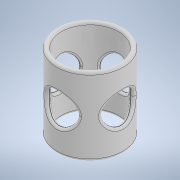
# Autodesk Inventor part: BlueYetiHolderSupport
Saved by Autodesk Inventor 2020 (Build 240168000, 168)
## iProperties
Created: 2020-08-02
Part Number: BlueYetiHolderSupport
Material: Generic
Document SubType Name: Sheet Metal
Designer: maple
Density: 1 g/cm^3
Sheet Metal Rule: Default
Appearance: Default
Author: maple
Autodesk Inventor part; units mm, degrees
ref_plane "YZ Plane" through (0, 0, 0) normal (1, 0, 0) x (0, 1, 0)
ref_plane "XZ Plane" through (0, 0, 0) normal (0, 1, 0) x (-1, 0, 0)
ref_plane "XY Plane" through (0, 0, 0) normal (0, 0, 1) x (1, 0, 0)
sketch "Sketch1" plane through (0, 0, 0) normal (0, 1, 0) x (-1, 0, 0)
  circle A0 centre (0, 0) radius 18.5
  line L0 (0, -18.5) -> (0, -21.5)
  circle A1 centre (0, 0) radius 21.5
  dimension "d0" = 37
  dimension "d1" = 3
  constraints: 2 coincident, 2 end point, 2 vertical alignment, 1 vertical, 4 other
  measures "d1" distance of L0.start L0.end
extrude "Extrusion1" add sketch "Sketch1" along normal blind 50
fillet "Fillet1" radius 1.5 4 edges at (18.5, 50, 0) (21.5, 50, 0) (18.5, 0, 0) (21.5, 0, 0)
sketch "Sketch2" plane through (0, 0, 0) normal (0, 0, 1) x (1, 0, 0)
  line L0 (0, 0) -> (0, 50)
  line L1 (-20, 50) -> (20, 50) projected
  circle A0 centre (0, 25) radius 10
  dimension "d5" = 20
  constraints: 2 end point, 2 midpoint, 1 centre point
  measures "d5" diameter of A0
extrude "Extrusion2" cut sketch "Sketch2" along normal mid plane 50
sketch "Sketch3" plane through (0, 0, 0) normal (1, 0, 0) x (0, 1, 0)
  line L0 (0, 0) -> (50.2134, 0)
  circle A0 centre (25.1067, 0) radius 10
  dimension "d8" = 20
  constraints: 2 end point, 1 centre point, 1 horizontal, 1 midpoint
  measures "d8" diameter of A0
extrude "Extrusion3" cut sketch "Sketch3" along normal mid plane 50
fillet "Fillet2" radius 1.4 10 edges at (-19.0329, 25.1117, -10) (-19.0329, 25.1016, 10) (21.4997, 15.1073, -0.1083) (-15.5644, 25.1001, 10) (-15.5644, 25.1133, -10) (18.4999, 15.1068, 0.0431) (-9.9997, 24.9282, 19.033) (-9.9997, 24.9282, -19.033) (-10, 25.007, 15.5644) (-10, 25.007, -15.5644)
equation "\"BendRadius\" = Thickness"
equation "\"BendReliefWidth\" = Thickness"
equation "\"BendReliefDepth\" = 0.5 * Thickness"
equation "\"CornerReliefSize\" = 4 * Thickness"
equation "\"MinimumRemnant\" = 2 * Thickness"
equation "\"TransitionRadius\" = BendRadius"
equation "\"JacobiRadiusSize\" = BendRadius"
equation "\"GapSize\" = Thickness"
equation "\"Thickness\" = 3.048"
body "Solid1"
